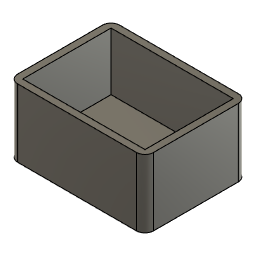
Enclosure_test1 (Autodesk Fusion 360 design; units mm, degrees)
Autodesk Fusion 360 part; units mm, degrees
box "BoxPrimitive1" add length 76.2 width 101.6 height 50.8 placed x (0, 0, -1) y (-1, 0, 0) z (0, 1, 0) at (101.6, 0, 63.5)
fillet "Fillet1" radius 6.35 1 edges at (101.6, 25.4, -12.7)
fillet "Fillet2" radius 6.35 1 edges at (101.6, 25.4, 63.5)
fillet "Fillet3" radius 6.35 1 edges at (0, 25.4, 63.5)
fillet "Fillet4" radius 6.35 1 edges at (0, 25.4, -12.7)
box "BoxPrimitive2" cut length 66.04 width 91.44 height -43.18 placed x (0, 0, 1) y (1, 0, 0) z (0, 1, 0) at (5.08, 50.8, -7.62)
shell "Shell1" thickness 3.175 removed faces 1 at (65.6167, 50.8, -9.3133)
cylinder "CylinderPrimitive1" add diameter 7.62 height 6.35 placed x (1, 0, 0) y (0, 0, -1) z (0, 1, 0) at (92.1502, 7.62, 53.9374)
hole "Hole1" at (92.1502, 13.97, 53.9374) direction (0, -1, 0) diameter 1.778 depth 5.08 tip angle 118
move_face "MoveFace1" by (-76.2, 0, 0) 1 faces at (94.9715, 13.97, 54.1489)
